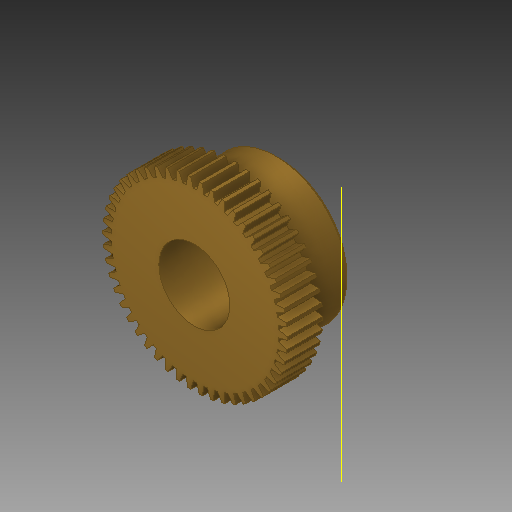
# Autodesk Inventor part: Schneckenrad
Saved by Autodesk Inventor 2019 (Build 230136000, 136)
## iProperties
Created: 2021-11-05
Part Number: Schneckenrad
Material: Messing, weicher Gelbton
Document SubType Name: Modeling
Designer: Bergi
Density: 8.47 g/cm^3
Appearance: Messing - satiniert
Mass: 30.8874 g
Surface Area: 24.5639 cm^2
Volume: 3.64669 cm^3
Author: Bergi
Autodesk Inventor part; units mm, degrees
ref_plane "XZ Plane" through (0, 0, 0) normal (0, 1, 0) x (-1, 0, 0)
ref_plane "XY Plane" through (0, 0, 0) normal (0, 0, 1) x (1, 0, 0)
sketch "Skizze1" plane through (0, 0, 0) normal (0, 0, 1) x (1, 0, 0)
  circle A0 centre (0, 0) radius 13
  dimension "d0" = 26
  constraints: 1 centre point, 1 coincident
  measures "d0" diameter of A0
extrude "Extrusion1" add sketch "Skizze1" along normal blind 5
sketch "Skizze2" plane through (0, 0, 5) normal (0, 0, 1) x (1, 0, 0)
  circle A0 centre (-0.1044, 0) radius 10
  point P0 (0, 0)
  dimension "d3" = 20
  constraints: 1 centre point
  measures "d3" diameter of A0
extrude "Extrusion2" add sketch "Skizze2" against normal blind 12
sketch "Skizze3" plane through (0, 0, 0) normal (0, 0, -1) x (-1, 0, 0)
  circle A0 centre (0, 0) radius 13 projected
  line L0 (-0.1962, 11.7904) -> (0.25, 11.7904)
  line L1 (0.25, 11.7904) -> (0.6, 12.9861)
  line L2 (0, -18.2) -> (0, 18.2) construction
  line L3 (-0.1962, 11.7904) -> (-0.25, 11.7904)
  line L4 (-0.25, 11.7904) -> (-0.6, 12.9861)
  arc A1 (0.6, 12.9861) -> (-0.6, 12.9861) centre (0, 0) ccw
  dimension "d6" = 0.5
  dimension "d7" = 1.2
  constraints: 8 end point, 2 horizontal alignment, 2 point on circle, 1 centre point, 1 coincident, 1 horizontal, 1 other
  measures "d6" distance of L0.end L3.end
  measures "d7" distance of L1.end L4.end
extrude "Extrusion3" cut sketch "Skizze3" against normal through all contours L1 L0 L3 L4 A0 picked at (0.0846, 12.1931)
pattern_circular "Runde Anordnung1" count 50 over 360 about axis through (0, 0, -10) along (0, 0, 1) of "Extrusion3"
sketch "Skizze4" plane through (-0.1044, 0, -7) normal (0, 0, -1) x (-1, 0, 0)
  circle A0 centre (0, 0) radius 10 projected
  circle A1 centre (0, 0) radius 5
  point P0 (-0.1044, 0)
  dimension "d13" = 10
  constraints: 1 centre point, 1 coincident
  measures "d13" diameter of A1
extrude "Extrusion4" cut sketch "Skizze4" against normal through all contours A1
chamfer "Fase1" distance 0.5 angle 45 1 edges at (-10.1044, 0, -7)
ref_plane "Arbeitsebene2" through (18.1871, 1.202, 0) normal (1, 0, 0) x (0, 1, 0)
ref_plane "Arbeitsebene1" through (12.3371, 1.202, 0) normal (1, 0, 0) x (0, 1, 0)
sketch "Skizze5" plane through (18.1871, 1.202, 0) normal (1, 0, 0) x (0, 1, 0)
  line L0 (-0.9854, 0) -> (-0.9854, 5) projected
  line L1 (-1.4186, 5) -> (-0.9854, 5) projected
  line L2 (-1.4186, 5) -> (-1.4186, 0) projected
  line L3 (-0.9854, 0) -> (-1.4186, 0) projected
  line L4 (-0.9854, 5) -> (-0.9854, 0) projected
  line L5 (-0.9854, 2.5) -> (15.5857, 2.5)
  point P0 (-1.202, 0)
  constraints: 2 end point, 1 horizontal, 1 midpoint
